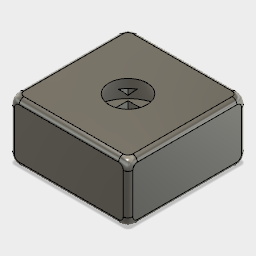
AdditivePrint (Autodesk Fusion 360 design; units mm, degrees)
Autodesk Fusion 360 part; units mm, degrees
sketch "Sketch1" plane through (0, 0, 0) normal (0, 1, 0) x (1, 0, 0)
  line L0 (0, 0) -> (6.35, 0)
  line L1 (6.35, 0) -> (6.35, 6.35)
  line L2 (6.35, 6.35) -> (0, 6.35)
  line L3 (0, 6.35) -> (0, 0)
  dimension "d3" = 6.35
  dimension "d4" = 6.35
  constraint horizontal L0
  constraint vertical L1
  constraint horizontal L2
  constraint vertical L3
  constraint coincident L0.start L3.end
  measures "d3" distance of L0.start
extrude "Extrude1" add sketch "Sketch1" along normal blind 3.175
ref_plane "WorkPlane1" through (3.175, 1.5875, -3.175) normal (0, 1, 0) x (0, 0, 1)
sketch "Sketch2" plane through (3.175, 1.5875, -3.175) normal (0, 1, 0) x (1, 0, 0)
  line L0 (-1.27, -1.27) -> (1.27, -1.27)
  line L1 (1.27, -1.27) -> (1.27, 1.27)
  line L2 (1.27, 1.27) -> (-1.27, 1.27)
  line L3 (-1.27, 1.27) -> (-1.27, -1.27)
  constraint horizontal L0
  constraint vertical L1
  constraint horizontal L2
  constraint vertical L3
extrude "Extrude2" cut sketch "Sketch2" along normal blind 0.7937 and the other way blind 0.7937
sketch "Sketch3" plane through (0, 3.175, 0) normal (0, 1, 0) x (-1, 0, 0)
  line L0 (0, -6.35) -> (0, 0)
  line L1 (0, 0) -> (-6.35, 0)
  line L2 (-6.35, 0) -> (-6.35, -6.35)
  line L3 (-6.35, -6.35) -> (0, -6.35)
  circle A0 centre (-3.175, -3.175) radius 1.016
  dimension "d9" = 2.032
  dimension "d10" = 3.175
  dimension "d11" = 3.175
  measures "d9" diameter of A0
  measures "d10" distance of L3
  measures "d11" distance of L0
extrude "Extrude3" cut sketch "Sketch3" against normal blind 1.5875 draft 30 contours A0
fillet "Fillet1" radius 0.254 12 edges at (0, 3.175, -3.175) (3.175, 3.175, 0) (0, 1.5875, 0) (3.175, 0, 0) (6.35, 1.5875, 0) (6.35, 0, -3.175) (6.35, 3.175, -3.175) (3.175, 3.175, -6.35) (6.35, 1.5875, -6.35) (3.175, 0, -6.35) (0, 1.5875, -6.35) (0, 0, -3.175)
equation "d5 = ( -0.125 / 2 ) * 1 in"
equation "d6 = ( 1 / 32 ) * 1 in"
equation "d7 = ( 1 / 32 ) * 1 in"
equation "d12 = ( -1 / 16 ) * 1 in"
